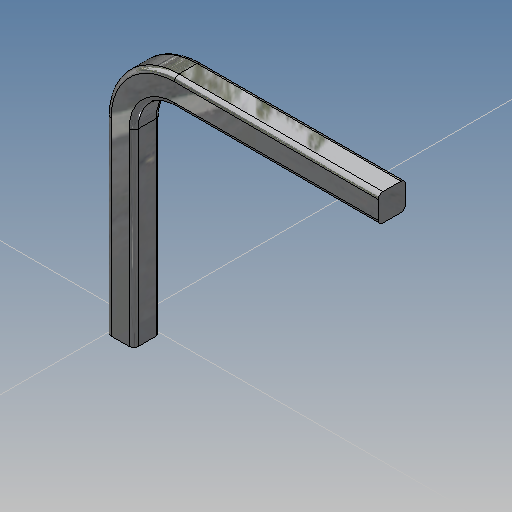
# Autodesk Inventor part: 90d pin_header
Saved by Autodesk Inventor 2019 (Build 230136000, 136)
## iProperties
Created: 2015-11-19
Part Number: 90d pin_header
Material: Allgemein
Document SubType Name: Modeling
Designer: Tom
Density: 1 g/cm^3
Appearance: Vorgabe
Mass: 0.00759062 g
Surface Area: 0.390327 cm^2
Volume: 0.00759062 cm^3
Author: Tom
Autodesk Inventor part; units mm, degrees
ref_plane "YZ Plane" through (0, 0, 0) normal (1, 0, 0) x (0, 1, 0)
ref_plane "XZ Plane" through (0, 0, 0) normal (0, 1, 0) x (-1, 0, 0)
ref_plane "XY Plane" through (0, 0, 0) normal (0, 0, 1) x (1, 0, 0)
sketch "Sketch1" plane through (0, 0, 0) normal (0, 0, 1) x (1, 0, 0)
  line L0 (7.62, 2.413) -> (1.905, 2.413)
  line L1 (0, 0.508) -> (0, 0)
  line L2 (0.762, 0) -> (0.762, 0.508)
  line L3 (1.905, 1.651) -> (7.62, 1.651)
  arc A0 (1.905, 1.651) -> (0.762, 0.508) centre (1.905, 0.508) ccw
  arc A1 (1.905, 2.413) -> (0, 0.508) centre (1.905, 0.508) ccw
  line L4 (7.62, 2.413) -> (7.62, 1.651)
  line L5 (0.762, 0) -> (0, 0)
  line L6 (0.762, -4.7752) -> (0, -4.7752)
  line L7 (0, -4.7752) -> (0, 0)
  line L8 (0, 0) -> (0.762, 0)
  line L9 (0.762, 0) -> (0.762, -4.7752)
  point P0 (0, 2.413)
  dimension "d0" = 7.62
  dimension "d1" = 0.762
  dimension "d2" = 1.143
  dimension "d3" = 1.905
  dimension "d4" = 2.413
  dimension "d5" = 4.7752
  constraints: 20 end point, 4 point on circle, 4 tangent, 3 perpendicular, 2 centre point, 2 parallel, 2 point on line, 1 horizontal
  measures "d0" distance of L0.start point (0, 2.413)
  measures "d1" distance between parallel lines of L0 L3
  measures "d2" radius of A0
  measures "d3" radius of A1
  measures "d4" distance from line of L1.end L0
  measures "d5" distance of L6.start L8.end
extrude "Extrusion1" add sketch "Sketch1" along normal blind 0.762
fillet "Fillet2" radius 0.127 8 edges at (1.0968, 1.3162, 0.762) (4.7625, 1.651, 0.762) (0.558, 1.855, 0.762) (4.7625, 2.413, 0.762) (0.558, 1.855, 0) (4.7625, 2.413, 0) (1.0968, 1.3162, 0) (4.7625, 1.651, 0)
body "Solid1"
